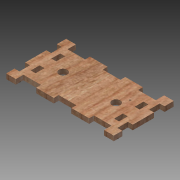
# Autodesk Inventor part: holder_plate
Saved by Autodesk Inventor 2014 SP1 (Build 180222100, 222)
## iProperties
Created: 2013-12-24
Part Number: holder_plate
Material: Wood (Birch)
Document SubType Name: Modeling
Designer: aoki
Density: 1 g/cm^3
Appearance: Birch - Natural Polished
Author: aoki
Autodesk Inventor part; units mm, degrees
ref_plane "YZ Plane" through (0, 0, 0) normal (1, 0, 0) x (0, 1, 0)
ref_plane "XZ Plane" through (0, 0, 0) normal (0, 1, 0) x (-1, 0, 0)
ref_plane "XY Plane" through (0, 0, 0) normal (0, 0, 1) x (1, 0, 0)
sketch "Block1" plane through (0, 0, 0) normal (0, 0, 1) x (1, 0, 0)
  line L0 (-30.1, 34.1) -> (-9.9, 34.1)
  line L1 (-9.9, 34.1) -> (-9.9, 25.1)
  line L2 (-9.9, 25.1) -> (9.9, 25.1)
  line L3 (9.9, 25.1) -> (9.9, 34.1)
  line L4 (9.9, 34.1) -> (30.1, 34.1)
  line L5 (30.1, 34.1) -> (30.1, 25.1)
  line L6 (30.1, 25.1) -> (49.9, 25.1)
  line L7 (49.9, 25.1) -> (49.9, 34.5715)
  line L8 (49.9, 34.5715) -> (61.1, 34.5715)
  line L9 (61.1, 34.5715) -> (61.1, 23.9)
  line L10 (61.1, 23.9) -> (52.1, 23.9)
  line L11 (52.1, 23.9) -> (52.1, 12.1)
  line L12 (52.1, 12.1) -> (61.1, 12.1)
  line L13 (61.1, 12.1) -> (61.1, -12.1)
  line L14 (61.1, -12.1) -> (52.1, -12.1)
  line L15 (52.1, -12.1) -> (52.1, -23.9)
  line L16 (52.1, -23.9) -> (61.1, -23.9)
  line L17 (61.1, -23.9) -> (61.1, -33.6285)
  line L18 (61.1, -33.6285) -> (49.9, -33.6285)
  line L19 (49.9, -33.6285) -> (49.9, -25.1)
  line L20 (49.9, -25.1) -> (30.1, -25.1)
  line L21 (30.1, -25.1) -> (30.1, -34.1)
  line L22 (30.1, -34.1) -> (9.9, -34.1)
  line L23 (9.9, -34.1) -> (9.9, -25.1)
  line L24 (9.9, -25.1) -> (-9.9, -25.1)
  line L25 (-9.9, -25.1) -> (-9.9, -34.1)
  line L26 (-9.9, -34.1) -> (-30.1, -34.1)
  line L27 (-30.1, -34.1) -> (-30.1, -25.1)
  line L28 (-30.1, -25.1) -> (-49.9, -25.1)
  line L29 (-49.9, -25.1) -> (-49.9, -33.6285)
  line L30 (-49.9, -33.6285) -> (-61.1, -33.6285)
  line L31 (-61.1, -33.6285) -> (-61.1, -23.9)
  line L32 (-61.1, -23.9) -> (-52.1, -23.9)
  line L33 (-52.1, -23.9) -> (-52.1, -12.1)
  line L34 (-52.1, -12.1) -> (-61.1, -12.1)
  line L35 (-61.1, -12.1) -> (-61.1, 12.1)
  line L36 (-61.1, 12.1) -> (-52.1, 12.1)
  line L37 (-52.1, 12.1) -> (-52.1, 23.9)
  line L38 (-52.1, 23.9) -> (-61.1, 23.9)
  line L39 (-61.1, 23.9) -> (-61.1, 34.5715)
  line L40 (-61.1, 34.5715) -> (-49.9, 34.5715)
  line L41 (-49.9, 34.5715) -> (-49.9, 25.1)
  line L42 (-49.9, 25.1) -> (-30.1, 25.1)
  line L43 (-30.1, 25.1) -> (-30.1, 34.1)
  line L44 (-40.9, 16.7667) -> (-50.1, 16.7667)
  line L45 (-50.1, 16.7667) -> (-50.1, 6.5667)
  line L46 (-50.1, 6.5667) -> (-40.9, 6.5667)
  line L47 (-40.9, 6.5667) -> (-40.9, 16.7667)
  line L48 (-40.9, -6.5667) -> (-50.1, -6.5667)
  line L49 (-50.1, -6.5667) -> (-50.1, -16.7667)
  line L50 (-50.1, -16.7667) -> (-40.9, -16.7667)
  line L51 (-40.9, -16.7667) -> (-40.9, -6.5667)
  circle A0 centre (-30, 0) radius 4.6
  circle A1 centre (30, 0) radius 4.6
  line L52 (50.1, 16.7667) -> (50.1, 6.5667)
  line L53 (50.1, 6.5667) -> (40.9, 6.5667)
  line L54 (40.9, 6.5667) -> (40.9, 16.7667)
  line L55 (40.9, 16.7667) -> (50.1, 16.7667)
  line L56 (50.1, -6.5667) -> (40.9, -6.5667)
  line L57 (40.9, -6.5667) -> (40.9, -16.7667)
  line L58 (40.9, -16.7667) -> (50.1, -16.7667)
  line L59 (50.1, -16.7667) -> (50.1, -6.5667)
  point P0 (0, 0.0615)
sketch "Block2" plane through (0, 0, 0) normal (0, 0, 1) x (1, 0, 0)
  line L0 (-30.2, 34.2) -> (-9.8, 34.2)
  line L1 (-9.8, 34.2) -> (-9.8, 25.2)
  line L2 (-9.8, 25.2) -> (9.8, 25.2)
  line L3 (9.8, 25.2) -> (9.8, 34.2)
  line L4 (9.8, 34.2) -> (30.2, 34.2)
  line L5 (30.2, 34.2) -> (30.2, 25.2)
  line L6 (30.2, 25.2) -> (49.8, 25.2)
  line L7 (49.8, 25.2) -> (49.8, 34.6715)
  line L8 (49.8, 34.6715) -> (61.2, 34.6715)
  line L9 (61.2, 34.6715) -> (61.2, 23.8)
  line L10 (61.2, 23.8) -> (52.2, 23.8)
  line L11 (52.2, 23.8) -> (52.2, 12.2)
  line L12 (52.2, 12.2) -> (61.2, 12.2)
  line L13 (61.2, 12.2) -> (61.2, -12.2)
  line L14 (61.2, -12.2) -> (52.2, -12.2)
  line L15 (52.2, -12.2) -> (52.2, -23.8)
  line L16 (52.2, -23.8) -> (61.2, -23.8)
  line L17 (61.2, -23.8) -> (61.2, -33.7285)
  line L18 (61.2, -33.7285) -> (49.8, -33.7285)
  line L19 (49.8, -33.7285) -> (49.8, -25.2)
  line L20 (49.8, -25.2) -> (30.2, -25.2)
  line L21 (30.2, -25.2) -> (30.2, -34.2)
  line L22 (30.2, -34.2) -> (9.8, -34.2)
  line L23 (9.8, -34.2) -> (9.8, -25.2)
  line L24 (9.8, -25.2) -> (-9.8, -25.2)
  line L25 (-9.8, -25.2) -> (-9.8, -34.2)
  line L26 (-9.8, -34.2) -> (-30.2, -34.2)
  line L27 (-30.2, -34.2) -> (-30.2, -25.2)
  line L28 (-30.2, -25.2) -> (-49.8, -25.2)
  line L29 (-49.8, -25.2) -> (-49.8, -33.7285)
  line L30 (-49.8, -33.7285) -> (-61.2, -33.7285)
  line L31 (-61.2, -33.7285) -> (-61.2, -23.8)
  line L32 (-61.2, -23.8) -> (-52.2, -23.8)
  line L33 (-52.2, -23.8) -> (-52.2, -12.2)
  line L34 (-52.2, -12.2) -> (-61.2, -12.2)
  line L35 (-61.2, -12.2) -> (-61.2, 12.2)
  line L36 (-61.2, 12.2) -> (-52.2, 12.2)
  line L37 (-52.2, 12.2) -> (-52.2, 23.8)
  line L38 (-52.2, 23.8) -> (-61.2, 23.8)
  line L39 (-61.2, 23.8) -> (-61.2, 34.6715)
  line L40 (-61.2, 34.6715) -> (-49.8, 34.6715)
  line L41 (-49.8, 34.6715) -> (-49.8, 25.2)
  line L42 (-49.8, 25.2) -> (-30.2, 25.2)
  line L43 (-30.2, 25.2) -> (-30.2, 34.2)
  circle A0 centre (-30, 0) radius 4.7
  circle A1 centre (30, 0) radius 4.7
  line L44 (50.2, 16.8667) -> (50.2, 6.4667)
  line L45 (50.2, 6.4667) -> (40.8, 6.4667)
  line L46 (40.8, 6.4667) -> (40.8, 16.8667)
  line L47 (40.8, 16.8667) -> (50.2, 16.8667)
  line L48 (50.2, -6.4667) -> (40.8, -6.4667)
  line L49 (40.8, -6.4667) -> (40.8, -16.8667)
  line L50 (40.8, -16.8667) -> (50.2, -16.8667)
  line L51 (50.2, -16.8667) -> (50.2, -6.4667)
  line L52 (-40.8, 16.8667) -> (-50.2, 16.8667)
  line L53 (-50.2, 16.8667) -> (-50.2, 6.4667)
  line L54 (-50.2, 6.4667) -> (-40.8, 6.4667)
  line L55 (-40.8, 6.4667) -> (-40.8, 16.8667)
  line L56 (-40.8, -6.4667) -> (-50.2, -6.4667)
  line L57 (-50.2, -6.4667) -> (-50.2, -16.8667)
  line L58 (-50.2, -16.8667) -> (-40.8, -16.8667)
  line L59 (-40.8, -16.8667) -> (-40.8, -6.4667)
  point P0 (0, 0.0615)
sketch "Block3" plane through (0, 0, 0) normal (0, 0, 1) x (1, 0, 0)
  line L0 (9.9, 34.1) -> (30.1, 34.1)
  line L1 (30.1, 34.1) -> (30.1, 25.1)
  line L2 (30.1, 25.1) -> (49.9, 25.1)
  line L3 (49.9, 25.1) -> (49.9, 34.5715)
  line L4 (49.9, 34.5715) -> (61.1, 34.5715)
  line L5 (61.1, 34.5715) -> (61.1, 23.9)
  line L6 (61.1, 23.9) -> (52.1, 23.9)
  line L7 (52.1, 23.9) -> (52.1, 12.1)
  line L8 (52.1, 12.1) -> (61.1, 12.1)
  line L9 (61.1, 12.1) -> (61.1, -12.1)
  line L10 (61.1, -12.1) -> (52.1, -12.1)
  line L11 (52.1, -12.1) -> (52.1, -23.9)
  line L12 (52.1, -23.9) -> (61.1, -23.9)
  line L13 (61.1, -23.9) -> (61.1, -33.6285)
  line L14 (61.1, -33.6285) -> (49.9, -33.6285)
  line L15 (49.9, -33.6285) -> (49.9, -25.1)
  line L16 (49.9, -25.1) -> (30.1, -25.1)
  line L17 (30.1, -25.1) -> (30.1, -34.1)
  line L18 (30.1, -34.1) -> (9.9, -34.1)
  line L19 (9.9, -34.1) -> (9.9, -25.1)
  line L20 (9.9, -25.1) -> (-9.9, -25.1)
  line L21 (-9.9, -25.1) -> (-9.9, -34.1)
  line L22 (-9.9, -34.1) -> (-30.1, -34.1)
  line L23 (-30.1, -34.1) -> (-30.1, -25.1)
  line L24 (-30.1, -25.1) -> (-49.9, -25.1)
  line L25 (-49.9, -25.1) -> (-49.9, -33.6285)
  line L26 (-49.9, -33.6285) -> (-61.1, -33.6285)
  line L27 (-61.1, -33.6285) -> (-61.1, -23.9)
  line L28 (-61.1, -23.9) -> (-52.1, -23.9)
  line L29 (-52.1, -23.9) -> (-52.1, -12.1)
  line L30 (-52.1, -12.1) -> (-61.1, -12.1)
  line L31 (-61.1, -12.1) -> (-61.1, 12.1)
  line L32 (-61.1, 12.1) -> (-52.1, 12.1)
  line L33 (-52.1, 12.1) -> (-52.1, 23.9)
  line L34 (-52.1, 23.9) -> (-61.1, 23.9)
  line L35 (-61.1, 23.9) -> (-61.1, 34.5715)
  line L36 (-61.1, 34.5715) -> (-49.9, 34.5715)
  line L37 (-49.9, 34.5715) -> (-49.9, 25.1)
  line L38 (-49.9, 25.1) -> (-30.1, 25.1)
  line L39 (-30.1, 25.1) -> (-30.1, 34.1)
  line L40 (-30.1, 34.1) -> (-9.9, 34.1)
  line L41 (-9.9, 34.1) -> (-9.9, 25.1)
  line L42 (-9.9, 25.1) -> (9.9, 25.1)
  line L43 (9.9, 25.1) -> (9.9, 34.1)
  circle A0 centre (-30, 0) radius 4.6
  circle A1 centre (30, 0) radius 4.6
  line L44 (-40.9, 16.7667) -> (-50.1, 16.7667)
  line L45 (-50.1, 16.7667) -> (-50.1, 6.5667)
  line L46 (-50.1, 6.5667) -> (-40.9, 6.5667)
  line L47 (-40.9, 6.5667) -> (-40.9, 16.7667)
  line L48 (-40.9, -6.5667) -> (-50.1, -6.5667)
  line L49 (-50.1, -6.5667) -> (-50.1, -16.7667)
  line L50 (-50.1, -16.7667) -> (-40.9, -16.7667)
  line L51 (-40.9, -16.7667) -> (-40.9, -6.5667)
  line L52 (50.1, 16.7667) -> (50.1, 6.5667)
  line L53 (50.1, 6.5667) -> (40.9, 6.5667)
  line L54 (40.9, 6.5667) -> (40.9, 16.7667)
  line L55 (40.9, 16.7667) -> (50.1, 16.7667)
  line L56 (50.1, -6.5667) -> (40.9, -6.5667)
  line L57 (40.9, -6.5667) -> (40.9, -16.7667)
  line L58 (40.9, -16.7667) -> (50.1, -16.7667)
  line L59 (50.1, -16.7667) -> (50.1, -6.5667)
  point P0 (0, 0.0615)
sketch "Block4" plane through (0, 0, 0) normal (0, 0, 1) x (1, 0, 0)
  line L0 (-30.08, 30.58) -> (-9.92, 30.58)
  line L1 (-9.92, 30.58) -> (-9.92, 25.08)
  line L2 (-9.92, 25.08) -> (9.92, 25.08)
  line L3 (9.92, 25.08) -> (9.92, 30.58)
  line L4 (9.92, 30.58) -> (30.08, 30.58)
  line L5 (30.08, 30.58) -> (30.08, 25.08)
  line L6 (30.08, 25.08) -> (49.92, 25.08)
  line L7 (49.92, 25.08) -> (49.92, 34.5515)
  line L8 (49.92, 34.5515) -> (61.08, 34.5515)
  line L9 (61.08, 34.5515) -> (61.08, 23.92)
  line L10 (61.08, 23.92) -> (55.58, 23.92)
  line L11 (55.58, 23.92) -> (55.58, 12.08)
  line L12 (55.58, 12.08) -> (61.08, 12.08)
  line L13 (61.08, 12.08) -> (61.08, -12.08)
  line L14 (61.08, -12.08) -> (55.58, -12.08)
  line L15 (55.58, -12.08) -> (55.58, -23.92)
  line L16 (55.58, -23.92) -> (61.08, -23.92)
  line L17 (61.08, -23.92) -> (61.08, -33.6085)
  line L18 (61.08, -33.6085) -> (49.92, -33.6085)
  line L19 (49.92, -33.6085) -> (49.92, -25.08)
  line L20 (49.92, -25.08) -> (30.08, -25.08)
  line L21 (30.08, -25.08) -> (30.08, -30.58)
  line L22 (30.08, -30.58) -> (9.92, -30.58)
  line L23 (9.92, -30.58) -> (9.92, -25.08)
  line L24 (9.92, -25.08) -> (-9.92, -25.08)
  line L25 (-9.92, -25.08) -> (-9.92, -30.58)
  line L26 (-9.92, -30.58) -> (-30.08, -30.58)
  line L27 (-30.08, -30.58) -> (-30.08, -25.08)
  line L28 (-30.08, -25.08) -> (-49.92, -25.08)
  line L29 (-49.92, -25.08) -> (-49.92, -33.6085)
  line L30 (-49.92, -33.6085) -> (-61.08, -33.6085)
  line L31 (-61.08, -33.6085) -> (-61.08, -23.92)
  line L32 (-61.08, -23.92) -> (-55.58, -23.92)
  line L33 (-55.58, -23.92) -> (-55.58, -12.08)
  line L34 (-55.58, -12.08) -> (-61.08, -12.08)
  line L35 (-61.08, -12.08) -> (-61.08, 12.08)
  line L36 (-61.08, 12.08) -> (-55.58, 12.08)
  line L37 (-55.58, 12.08) -> (-55.58, 23.92)
  line L38 (-55.58, 23.92) -> (-61.08, 23.92)
  line L39 (-61.08, 23.92) -> (-61.08, 34.5515)
  line L40 (-61.08, 34.5515) -> (-49.92, 34.5515)
  line L41 (-49.92, 34.5515) -> (-49.92, 25.08)
  line L42 (-49.92, 25.08) -> (-30.08, 25.08)
  line L43 (-30.08, 25.08) -> (-30.08, 30.58)
  line L44 (-44.42, 16.7467) -> (-50.08, 16.7467)
  line L45 (-50.08, 16.7467) -> (-50.08, 6.5867)
  line L46 (-50.08, 6.5867) -> (-44.42, 6.5867)
  line L47 (-44.42, 6.5867) -> (-44.42, 16.7467)
  line L48 (-44.42, -6.5867) -> (-50.08, -6.5867)
  line L49 (-50.08, -6.5867) -> (-50.08, -16.7467)
  line L50 (-50.08, -16.7467) -> (-44.42, -16.7467)
  line L51 (-44.42, -16.7467) -> (-44.42, -6.5867)
  circle A0 centre (-30, 0) radius 4.83
  circle A1 centre (30, 0) radius 4.83
  line L52 (50.08, 16.7467) -> (50.08, 6.5867)
  line L53 (50.08, 6.5867) -> (44.42, 6.5867)
  line L54 (44.42, 6.5867) -> (44.42, 16.7467)
  line L55 (44.42, 16.7467) -> (50.08, 16.7467)
  line L56 (50.08, -6.5867) -> (44.42, -6.5867)
  line L57 (44.42, -6.5867) -> (44.42, -16.7467)
  line L58 (44.42, -16.7467) -> (50.08, -16.7467)
  line L59 (50.08, -16.7467) -> (50.08, -6.5867)
  point P0 (0, 0.0615)
sketch "Sketch10" plane through (0, 0, 0) normal (0, 0, 1) x (1, 0, 0)
  line L0 (50, -25) -> (-50, -25)
  line L1 (-50, -25) -> (-50, 25)
  line L2 (-50, 25) -> (50, 25)
  line L3 (50, 25) -> (50, -25)
  line L4 (50, -25) -> (-50, 25) construction
  line L5 (-50, -25) -> (50, 25) construction
  point P0 (0, 0)
  dimension "d21" = 100
  dimension "d22" = 50
  constraints: 12 end point, 2 midpoint, 2 parallel, 1 horizontal, 1 perpendicular
  measures "d21" distance of L1.end L2.end
  measures "d22" distance of L0.end L1.end
extrude "Extrusion2" add sketch "Sketch10" against normal blind 5.5
sketch "Sketch16" plane through (0, 0, -5.5) normal (0, 0, -1) x (-1, 0, 0)
  line L0 (0, -48.2244) -> (0, 50.6464) projected
  point P0 (0, 0)
  point P1 (-30, 0)
  point P2 (30, 0)
  dimension "d52" = 60
  constraints: 1 symmetric about line
  measures "d52" distance of point (30, 0) point (-30, 0)
hole "Hole5" at (30, 0, -5.5) at (-30, 0, -5.5) direction (0, 0, 1) diameter 9.5 end through all
sketch "Sketch35" plane through (0, 0, 0) normal (0, 0, 1) x (1, 0, 0)
  line L0 (-50, 25) -> (50, 25) projected
  line L1 (-50, -25) -> (-50, 25) projected
  line L2 (0, -48.2244) -> (0, 50.6464) projected
  line L3 (-246.2787, 0) -> (113.734, 0) projected
  line L4 (50, 25) -> (50, -25) projected
  line L5 (-30, 25) -> (-30, 30.5)
  line L6 (-30, 30.5) -> (-10, 30.5)
  line L7 (-10, 30.5) -> (-10, 25)
  line L8 (-30, 25) -> (-10, 25)
  line L9 (30, 25) -> (30, 30.5)
  line L10 (30, 30.5) -> (10, 30.5)
  line L11 (10, 30.5) -> (10, 25)
  line L12 (30, 25) -> (10, 25)
  line L13 (-30, -25) -> (-30, -30.5)
  line L14 (-30, -30.5) -> (-10, -30.5)
  line L15 (-10, -30.5) -> (-10, -25)
  line L16 (-30, -25) -> (-10, -25)
  line L17 (30, -25) -> (30, -30.5)
  line L18 (30, -25) -> (10, -25)
  line L19 (30, -30.5) -> (10, -30.5)
  line L20 (10, -30.5) -> (10, -25)
  point P0 (0, 0)
  point P1 (-50, 16.6667)
  point P2 (-50, 4.1667)
  dimension "d129" = 20
  dimension "d130" = 20
  dimension "d131" = 5.5
  constraints: 32 end point, 18 symmetric about line, 6 point on line, 3 perpendicular, 1 parallel
  measures "d129" distance between parallel lines of L5 L1
  measures "d130" distance of L5.end L6.end
  measures "d131" distance of L6.end L7.end
extrude "Extrusion6" add sketch "Sketch35" against normal blind 5.5 contours L5 L6 L7 L0 | L11 L10 L9 L0 | L16 L15 L14 L13 | L17 L19 L20 L18
sketch "Sketch36" plane through (0, 0, 0) normal (0, 0, 1) x (1, 0, 0)
  line L0 (-50, 25) -> (-30, 25) projected
  line L1 (-50, -25) -> (-50, 25) projected
  line L2 (-50, 16.6667) -> (-44.5, 16.6667)
  line L3 (-44.5, 16.6667) -> (-44.5, 6.6667)
  line L4 (-44.5, 6.6667) -> (-50, 6.6667)
  line L5 (-50, 6.6667) -> (-50, 16.6667)
  line L6 (-246.2787, 0) -> (113.734, 0) projected
  line L7 (0, -48.2244) -> (0, 50.6464) projected
  line L8 (-50, -16.6667) -> (-44.5, -16.6667)
  line L9 (-44.5, -16.6667) -> (-44.5, -6.6667)
  line L10 (-44.5, -6.6667) -> (-50, -6.6667)
  line L11 (-50, -6.6667) -> (-50, -16.6667)
  line L12 (50, 16.6667) -> (44.5, 16.6667)
  line L13 (44.5, 16.6667) -> (44.5, 6.6667)
  line L14 (44.5, 6.6667) -> (50, 6.6667)
  line L15 (50, 6.6667) -> (50, 16.6667)
  line L16 (44.5, -16.6667) -> (44.5, -6.6667)
  line L17 (44.5, -6.6667) -> (50, -6.6667)
  line L18 (50, -6.6667) -> (50, -16.6667)
  line L19 (50, -16.6667) -> (44.5, -16.6667)
  point P0 (0, 0)
  dimension "d144" = 5.5
  dimension "d145" = 10
  dimension "d146" = 8.3333
  constraints: 32 end point, 12 symmetric about line, 2 parallel, 1 horizontal, 1 perpendicular, 1 point on line
  measures "d144" distance of L2.start L2.end
  measures "d145" distance of L2.end L3.end
  measures "d146" distance between parallel lines of L0 L2
extrude "Extrusion7" cut sketch "Sketch36" against normal through all
sketch "Sketch37" plane through (0, 0, 0) normal (0, 0, 1) x (1, 0, 0)
  line L0 (30, -30.5) -> (10, -30.5)
  line L1 (-10, -30.5) -> (-30, -30.5)
  line L2 (0, -48.2244) -> (0, 50.6464) projected
  line L3 (-50, 34.4715) -> (-61, 34.4715)
  line L4 (-61, 34.4715) -> (-61, -33.5285)
  line L5 (-61, -33.5285) -> (-50, -33.5285)
  line L6 (-50, -33.5285) -> (-50, 34.4715)
  line L7 (50, 16.6667) -> (50, 25)
  line L8 (50, -6.6667) -> (50, 6.6667)
  line L9 (50, -25) -> (50, -16.6667)
  line L10 (50, 34.4715) -> (61, 34.4715)
  line L11 (61, 34.4715) -> (61, -33.5285)
  line L12 (61, -33.5285) -> (50, -33.5285)
  line L13 (50, -33.5285) -> (50, 34.4715)
  point P0 (0, 0)
  dimension "d155" = 11
  constraints: 26 end point, 4 symmetric about line, 2 parallel, 1 horizontal, 1 perpendicular
  measures "d155" distance of L5.end L4.end
extrude "Extrusion8" add sketch "Sketch37" against normal blind 5.5
sketch "Sketch38" plane through (0, 0, 0) normal (0, 0, 1) x (1, 0, 0)
  line L0 (-61, 34.4715) -> (-61, -33.5285) projected
  line L1 (-246.2787, 0) -> (113.734, 0) projected
  line L2 (0, -48.2244) -> (0, 50.6464) projected
  line L3 (-61, 12) -> (-55.5, 12)
  line L4 (-55.5, 12) -> (-55.5, 24)
  line L5 (-55.5, 24) -> (-61, 24)
  line L6 (-61, 24) -> (-61, 12)
  line L7 (-61, -12) -> (-55.5, -12)
  line L8 (-55.5, -12) -> (-55.5, -24)
  line L9 (-55.5, -24) -> (-61, -24)
  line L10 (-61, -24) -> (-61, -12)
  line L11 (61, 12) -> (55.5, 12)
  line L12 (55.5, 12) -> (55.5, 24)
  line L13 (55.5, 24) -> (61, 24)
  line L14 (61, 24) -> (61, 12)
  line L15 (55.5, -12) -> (55.5, -24)
  line L16 (55.5, -24) -> (61, -24)
  line L17 (61, -24) -> (61, -12)
  line L18 (61, -12) -> (55.5, -12)
  point P0 (0, 0)
  dimension "d164" = 5.5
  dimension "d165" = 12
  dimension "d166" = 12
  constraints: 32 end point, 12 symmetric about line, 2 parallel, 1 horizontal, 1 perpendicular, 1 point on line
  measures "d164" distance of L5.end L4.end
  measures "d165" distance of L4.end L3.end
  measures "d166" distance between parallel lines of L1 L3
extrude "Extrusion10" cut sketch "Sketch38" against normal through all
equation "\"d23\" = Wt"
equation "\"d129\" = 0.2 * d21"
equation "\"d130\" = 0.2 * d21"
equation "\"d131\" = Wt"
equation "\"d142\" = Wt"
equation "\"d144\" = Wt"
equation "\"d145\" = 0.2 * d22"
equation "\"d146\" = 0.166667 * d22"
equation "\"d147\" = Wt"
equation "\"d162\" = Wt"
equation "\"d164\" = Wt"
equation "\"d172\" = Wt"
equation "\"Wt\" = 5.5"
body "Solid2"
